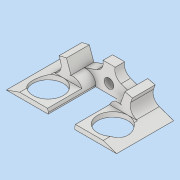
# Autodesk Inventor part: aftPotentiometerMount
Saved by Autodesk Inventor 2017 (Build 210142000, 142)
## iProperties
Created: 2016-12-12
Part Number: aftPotentiometerMount
Material: ABS Plastic
Document SubType Name: Modeling
Designer: techn
Density: 1.06 g/cm^3
Appearance: Smooth - White
Author: techn
Autodesk Inventor part; units mm, degrees
ref_plane "YZ Plane" through (0, 0, 0) normal (1, 0, 0) x (0, 1, 0)
ref_plane "XZ Plane" through (0, 0, 0) normal (0, 1, 0) x (-1, 0, 0)
ref_plane "XY Plane" through (0, 0, 0) normal (0, 0, 1) x (1, 0, 0)
sketch "Sketch1" plane through (0, 0, 0) normal (0, 0, 1) x (1, 0, 0)
  circle A0 centre (0, 0) radius 47.625
  line L0 (0, 0) -> (0, 41.91)
  circle A1 centre (0, 41.91) radius 1.5875
  line L1 (-10.795, 38.735) -> (10.795, 38.735)
  circle A2 centre (0, 41.91) radius 3.175
  line L2 (-10.795, 38.735) -> (-18.415, 38.735)
  line L3 (10.795, 38.735) -> (18.415, 38.735)
  line L4 (18.415, 38.735) -> (1.0632, 44.9017)
  line L5 (-18.415, 38.735) -> (-1.0632, 44.9017)
  line L6 (-1.0632, 44.9017) -> (-2.0159, 47.5823)
  line L7 (1.0632, 44.9017) -> (2.0159, 47.5823)
  line L8 (8.2433, 42.35) -> (9.7588, 46.6144)
  line L9 (10.6366, 41.4994) -> (12.2446, 46.024)
  line L10 (-8.2433, 42.35) -> (-9.7588, 46.6144)
  line L11 (-10.6366, 41.4994) -> (-12.2446, 46.024)
  dimension "d0" = 95.25
  dimension "d1" = 41.91
  dimension "d2" = 3.175
  dimension "d3" = 21.59
  dimension "d4" = 3.175
  dimension "d5" = 10.795
  dimension "d6" = 6.35
  dimension "d7" = 7.62
  dimension "d8" = 7.62
  dimension "d27" = 7.62
  dimension "d28" = 2.54
  dimension "d29" = 7.62
  dimension "d30" = 2.54
  constraints: 24 end point, 8 point on circle, 5 perpendicular, 4 point on line, 3 centre point, 3 coincident, 3 horizontal, 2 tangent, 1 parallel, 1 vertical
  measures "d0" diameter of A0
  measures "d1" distance of L0.start L0.end
  measures "d2" diameter of A1
  measures "d3" distance of L1.start L1.end
  measures "d4" distance from line of L0.end L1
  measures "d5" horizontal distance of L0.end L1.start
  measures "d6" diameter of A2
  measures "d7" distance of L1.start L2.end
  measures "d8" distance of L1.end L3.end
  measures "d27" distance of L4.end L8.start
  measures "d28" distance of L8.start L9.start
  measures "d29" distance of L10.start L5.end
  measures "d30" distance of L11.start L10.start
extrude "Extrusion1" add sketch "Sketch1" along normal blind 3.175 contours L4 L3 L1 A2 | L5 A2 L1 L2 | L7 A2 L6 A0 | A2
sketch "Sketch2" plane through (0, 0, 3.175) normal (0, 0, 1) x (1, 0, 0)
  circle A0 centre (0, 41.91) radius 1.5875 projected
  line L0 (-1.0632, 44.9017) -> (-18.415, 38.735) projected
  line L1 (-18.415, 38.735) -> (18.415, 38.735) projected
  line L2 (18.415, 38.735) -> (1.0632, 44.9017) projected
  line L3 (1.0632, 44.9017) -> (2.0159, 47.5823) projected
  arc A1 (2.0159, 47.5823) -> (-2.0159, 47.5823) centre (0, 0) ccw projected
  line L4 (-2.0159, 47.5823) -> (-1.0632, 44.9017) projected
  line L5 (-4.445, 38.735) -> (-4.445, 43.6998)
  line L6 (-18.415, 38.735) -> (18.415, 38.735) projected
  line L7 (4.445, 38.735) -> (4.445, 43.6998)
  dimension "d11" = 13.97
  constraints: 4 end point, 4 point on line, 2 parallel, 1 vertical
  measures "d11" distance from line of L5 L0.end
extrude "Extrusion2" add sketch "Sketch2" along normal blind 15.875 contours L5 L1 L0 | L7 L2 L1
sketch "Sketch3" plane through (-18.415, 38.735, 0) normal (0, -1, 0) x (1, 0, 0)
  line L0 (0, 0) -> (36.83, 0) projected
  line L1 (36.83, 0) -> (36.83, 19.05) projected
  line L2 (22.86, 19.05) -> (36.83, 19.05) projected
  line L3 (22.86, 3.175) -> (22.86, 19.05) projected
  line L4 (13.97, 3.175) -> (22.86, 3.175) projected
  line L5 (13.97, 3.175) -> (13.97, 19.05) projected
  line L6 (0, 19.05) -> (13.97, 19.05) projected
  line L7 (0, 0) -> (0, 19.05) projected
  circle A0 centre (7.62, 12.7) radius 5.08
  circle A1 centre (29.21, 12.7) radius 5.08
  point P0 (18.415, 0)
  dimension "d14" = 10.16
  dimension "d15" = 10.16
  dimension "d16" = 6.35
  dimension "d17" = 6.35
  dimension "d18" = 6.35
  dimension "d19" = 6.35
  constraints: 2 centre point
  measures "d14" diameter of A0
  measures "d15" diameter of A1
  measures "d16" distance from line of L3 A1.centre
  measures "d17" distance from line of L5 A0.centre
  measures "d18" distance from line of L6 A0.centre
  measures "d19" distance from line of L2 A1.centre
extrude "Extrusion3" cut sketch "Sketch3" against normal blind 12.7 contours A0 | A1
ref_plane "Work Plane1" through (-18.415, 40.3225, 0) normal (0, -1, 0) x (1, 0, 0)
sketch "Sketch4" plane through (-18.415, 40.3225, 0) normal (0, -1, 0) x (1, 0, 0)
  circle A0 centre (29.21, 12.7) radius 5.08 projected
  line L0 (36.83, 0) -> (19.4782, 0) projected
  line L1 (19.4782, 0) -> (19.4782, 3.175) projected
  line L2 (22.86, 3.175) -> (19.4782, 3.175) projected
  line L3 (22.86, 3.175) -> (22.86, 19.05) projected
  line L4 (36.83, 19.05) -> (22.86, 19.05) projected
  line L5 (36.83, 0) -> (36.83, 19.05) projected
  circle A1 centre (7.62, 12.7) radius 5.08 projected
  line L6 (17.3518, 0) -> (0, 0) projected
  line L7 (0, 0) -> (0, 19.05) projected
  line L8 (13.97, 19.05) -> (0, 19.05) projected
  line L9 (13.97, 3.175) -> (13.97, 19.05) projected
  line L10 (17.3518, 3.175) -> (13.97, 3.175) projected
  line L11 (17.3518, 0) -> (17.3518, 3.175) projected
  line L12 (36.83, 19.05) -> (22.86, 19.05) projected
  line L13 (36.83, 19.05) -> (22.86, 19.05)
  line L14 (22.86, 19.05) -> (22.86, 7.62)
  line L15 (22.86, 7.62) -> (36.83, 7.62)
  line L16 (36.83, 7.62) -> (36.83, 19.05)
  line L17 (0, 19.05) -> (13.97, 19.05)
  line L18 (13.97, 19.05) -> (13.97, 7.62)
  line L19 (13.97, 7.62) -> (0, 7.62)
  line L20 (0, 7.62) -> (0, 19.05)
  circle A2 centre (29.21, 12.7) radius 5.08 projected
  circle A3 centre (7.62, 12.7) radius 5.08 projected
  point P0 (18.415, 0)
  constraints: 16 end point, 4 parallel, 2 horizontal, 2 perpendicular, 2 point on line, 2 tangent
extrude "Extrusion4" cut sketch "Sketch4" against normal blind 12.7 contours A0 | L15 L3 L4 L5 | A1 | L19 L7 L8 L9
fillet "Fillet1" radius 3.175 2 edges at (1.0632, 44.9017, 1.5875) (-1.0632, 44.9017, 1.5875)
fillet "Fillet2" radius 3.175 2 edges at (-4.445, 43.6998, 5.3975) (4.445, 43.6998, 5.3975)
extrude "Extrusion5" add sketch "Sketch1" along normal up to surface (7.62 mm away) contours L9 L4 L8 A0 | A0 L10 L5 L11
fillet "Fillet3" radius 3.175 2 edges at (-10.6366, 41.4994, 3.81) (10.6366, 41.4994, 3.81)
equation "\"d5\" = 0.5 * d3"
body "Solid1"
